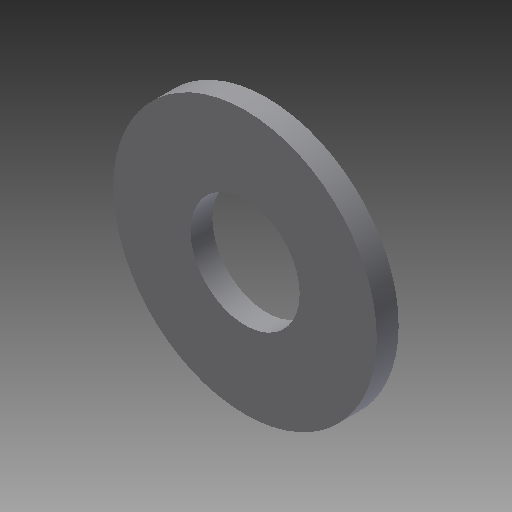
# Autodesk Inventor part: 4489_washer
Saved by Autodesk Inventor 2019 (Build 230136000, 136)
## iProperties
Category: PARTsolutions
Company: 8020
Created: 2019-03-04
Part Number: 4489_washer
Material: Generic
Catalog Web Link: www.cadenas.de
Description: 4488, 4489_washer-Combination Hinges
Vendor: 8020
Document SubType Name: Modeling
Designer: psadmin
Manufacturer: 8020
Mass: 0.425842 g
Surface Area: 6.61964 cm^2
Volume: 0.425842 cm^3
Density: 1 g/cm^3
Appearance: PSOLRGB-192-192-192
PSOL_IDENT_0: {$CADENAS_DATA\23d-libs\8020\inch\panels_and_doors\4488_washer.prj},174 {VTYP=3D},{NB=4489_washer},{
PSOL_IDENT_1: LINA=4489_washer},{NN=4488, 4489_washer},{DATE=04.12.2018 10:30:19},{GEOMDATE=14.12.2011 08:55:00},{
PSOL_IDENT_2: VERSION=},{LINEID=320},{WBVAR=},{WBNUMERIC=}  {NB=4489_washer},{LINA=4489_washer},{KT=DUMMY},{PN=448
PSOL_IDENT_3: 9}
NN: 4488, 4489_washer
NT: Combination Hinges
NB: 4489_washer
NBSYN: $PN._washer
LINA: 4489_washer
PN: 4489
SUPPLIER: 8020
ARTICLENO: 4489_washer
BOMINFO: 4489_washer
CREATOR: CADENAS GmbH
Title: 4489_washer
Author: Cadenas PARTsolutions
Comments: Combination Hinges
Autodesk Inventor part; units mm, degrees
sketch "Sketch_1" plane through (0, 0, 0) normal (0, 0, 1) x (1, 0, 0)
  circle A0 centre (0, 0) radius 9.9568
  circle A1 centre (0, 0) radius 4.1275
  constraints: 2 centre point
extrude "Extrusion1" add sketch "Sketch_1" along normal blind 1.651
ref_plane "to_a_XY" through (0, 0, 0) normal (0, 0, 1) x (1, 0, 0)
ref_plane "to_a_YZ" through (0, 0, 0) normal (1, 0, 0) x (0, 1, 0)
ref_plane "to_a_ZX" through (0, 0, 0) normal (0, 1, 0) x (0, 0, 1)
body "Solid1"
